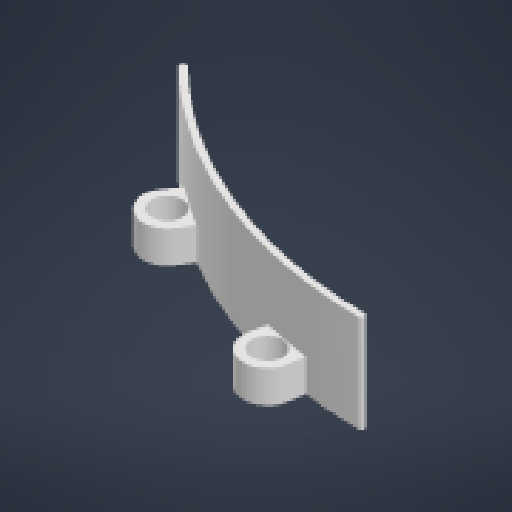
# Autodesk Inventor part: wall_standard
Saved by Autodesk Inventor 2026 (Build 300175050, 175E)
## iProperties
Created: 2026-04-30
Part Number: wall_standard
Material: Generic
Document SubType Name: Modeling
Designer: sniel
Density: 1 g/cm^3
Appearance: Default
Author: sniel
Autodesk Inventor part; units mm, degrees
ref_plane "YZ Plane" through (0, 0, 0) normal (1, 0, 0) x (0, 1, 0)
ref_plane "XZ Plane" through (0, 0, 0) normal (0, 1, 0) x (-1, 0, 0)
ref_plane "XY Plane" through (0, 0, 0) normal (0, 0, 1) x (1, 0, 0)
sketch "Sketch1" plane through (0, 0, 0) normal (0, 1, 0) x (-1, 0, 0)
  circle A0 centre (26.4627, 138.7343) radius 5
  circle A1 centre (79.388, 116.8119) radius 5
  arc A2 (96.3331, 96.3331) -> (82.5566, 108.3722) centre (0, 0) ccw
  line L0 (82.5566, 108.3722) -> (85.4769, 112.4329)
  arc A3 (85.4769, 112.4329) -> (73.0752, 120.8614) centre (79.388, 116.8119) ccw
  line L1 (73.0752, 120.8614) -> (70.3746, 116.6514)
  arc A4 (70.3746, 116.6514) -> (32.7226, 132.2473) centre (0, 0) ccw
  line L2 (32.7226, 132.2473) -> (33.7899, 137.1339)
  arc A5 (33.7899, 137.1339) -> (19.0608, 139.9434) centre (26.4627, 138.7343) ccw
  line L3 (19.0608, 139.9434) -> (18.2544, 135.007)
  arc A6 (18.2544, 135.007) -> (0, 136.2355) centre (0, 0) ccw
  line L4 (0, 136.2355) -> (0, 134.2355)
  arc A7 (94.9189, 94.9189) -> (0, 134.2355) centre (0, 0) ccw
  line L5 (94.9189, 94.9189) -> (96.3331, 96.3331)
  constraints: 12 end point, 12 point on circle, 8 centre point
extrude "Extrusion1" add sketch "Sketch1" along normal blind 30 contours A0 | A1 | L5 A7 L4 A6 L3 A5 L2 A4 L1 A3 L0 A2
sketch "Sketch2" plane through (0, 30, 0) normal (0, 1, 0) x (1, 0, 0)
  arc A0 (-96.3331, -96.3331) -> (-82.5566, -108.3722) centre (0, 0) ccw projected
  line L0 (-82.5566, -108.3722) -> (-85.4769, -112.4329) projected
  arc A1 (-85.4769, -112.4329) -> (-73.0752, -120.8614) centre (-79.388, -116.8119) ccw projected
  line L1 (-73.0752, -120.8614) -> (-70.3746, -116.6514) projected
  arc A2 (-70.3746, -116.6514) -> (-32.7226, -132.2473) centre (0, 0) ccw projected
  line L2 (-32.7226, -132.2473) -> (-33.7899, -137.1339) projected
  arc A3 (-33.7899, -137.1339) -> (-19.0608, -139.9434) centre (-26.4627, -138.7343) ccw projected
  line L3 (-19.0608, -139.9434) -> (-18.2544, -135.007) projected
  arc A4 (-18.2544, -135.007) -> (0, -136.2355) centre (0, 0) ccw projected
  line L4 (0, -136.2355) -> (0, -134.2355) projected
  arc A5 (-94.9189, -94.9189) -> (0, -134.2355) centre (0, 0) ccw projected
  line L5 (-94.9189, -94.9189) -> (-96.3331, -96.3331) projected
  circle A6 centre (0, 0) radius 136.2355
  point P0 (0, 0)
  point P1 (-82.5566, -108.3722)
  constraints: 1 coincident, 3 other
extrude "Extrusion2" cut sketch "Sketch2" against normal blind 20 contours A6 L1 A1 L0 | A6 L3 A3 L2
sketch "Sketch3" plane through (0, 0, 0) normal (0, -1, 0) x (1, 0, 0)
  arc A0 (-82.5566, 108.3722) -> (-96.3331, 96.3331) centre (0, 0) ccw projected
  line L0 (-94.9189, 94.9189) -> (-96.3331, 96.3331) projected
  arc A1 (0, 134.2355) -> (-94.9189, 94.9189) centre (0, 0) ccw projected
  line L1 (0, 136.2355) -> (0, 134.2355) projected
  arc A2 (0, 136.2355) -> (-18.2544, 135.007) centre (0, 0) ccw projected
  line L2 (-19.0608, 139.9434) -> (-18.2544, 135.007) projected
  arc A3 (-19.0608, 139.9434) -> (-33.7899, 137.1339) centre (-26.4627, 138.7343) ccw projected
  line L3 (-32.7226, 132.2473) -> (-33.7899, 137.1339) projected
  arc A4 (-32.7226, 132.2473) -> (-70.3746, 116.6514) centre (0, 0) ccw projected
  line L4 (-73.0752, 120.8614) -> (-70.3746, 116.6514) projected
  arc A5 (-73.0752, 120.8614) -> (-85.4769, 112.4329) centre (-79.388, 116.8119) ccw projected
  line L5 (-82.5566, 108.3722) -> (-85.4769, 112.4329) projected
  circle A6 centre (-26.4627, 138.7343) radius 4.75
  circle A7 centre (-79.388, 116.8119) radius 4.75
  point P0 (0, 0)
  dimension "d7" = 9.5
  dimension "d8" = 9.5
  constraints: 2 centre point, 2 coincident
  measures "d7" diameter of A6
  measures "d8" diameter of A7
extrude "Extrusion3" cut sketch "Sketch3" against normal blind 10 contours A6 | A7
fillet "Fillet1" radius 1 4 edges at (0, 15, 136.2355) (0, 15, 134.2355) (-96.3331, 15, 96.3331) (-94.9189, 15, 94.9189)
body "Solid1"
